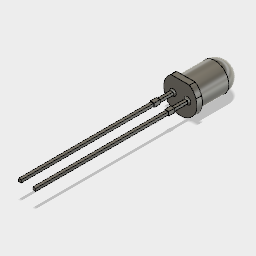
Diode with cutout v1 (Autodesk Fusion 360 design; units mm, degrees)
Autodesk Fusion 360 part; units mm, degrees
cylinder "CylinderPrimitive1" add diameter 5 height 0.5 placed x (1, 0, 0) y (0, 1, 0) z (0, 0, 1) at (0, 0, 0) makes body 1
move_body "Move1" bodies 1 to x (1, 0, 0) y (0, 1, 0) z (0, 0, 1) at (-2.2514, 0, -0.3716)
move_face "MoveFace1" by (0, 0, -4.6246) 1 faces at (-3.1377, 0.2321, -0.3716) on bodies 1
sphere "SpherePrimitive1" add diameter 5 placed x (1, 0, 0) y (0, 0, -1) z (0, 1, 0) at (-2.2514, 0, -4.9962) bodies 1
cylinder "CylinderPrimitive2" add diameter 5.9 height 1 placed x (1, 0, 0) y (0, 1, 0) z (0, 0, 1) at (6.2604, 2.0707, 0.1284) separate body makes body 2
move_body "Move2" bodies 2 to x (1, 0, 0) y (0, 1, 0) z (0, 0, 1) at (-8.4959, 0, 0)
move_body "Move3" bodies 2 to x (1, 0, 0) y (0, 1, 0) z (0, 0, 1) at (-0.0535, -1.9528, 0)
cylinder "CylinderPrimitive3" add diameter 5.906 height 1 placed x (1, 0, 0) y (0, 1, 0) z (0, 0, 1) at (-2.2514, 0, 0.1284) bodies 1
combine "Combine1" operation add target body 2 tool bodies 1
sphere "SpherePrimitive2" add diameter 1.5 placed x (1, 0, 0) y (0, 0, -1) z (0, 1, 0) at (-3.6739, 0, 2.7436) separate body makes body 3
move_body "Move4" bodies 3 to x (1, 0, 0) y (0, 1, 0) z (0, 0, 1) at (0.1106, 0, -2.102)
copy_body "CopyPasteBodies1" bodies 3 makes body 4
move_body "Move5" bodies 4 to x (1, 0, 0) y (0, 1, 0) z (0, 0, 1) at (2.5576, 0, 0.0489)
combine "Combine2" operation add target body 2 tool bodies 3 4
box "BoxPrimitive1" add length 27 width 0.5 height 0.5 placed x (0, 0, 1) y (1, 0, 0) z (0, 1, 0) at (-3.8323, 0, 1.4941) separate body makes body 5
move_body "Move6" bodies 5 to x (1, 0, 0) y (0, 1, 0) z (0, 0, 1) at (-0.0201, -0.2558, -0.183)
move_body "Move7" bodies 5 to x (1, 0, 0) y (0, 1, 0) z (0, 0, 1) at (0.0552, 0, 0.0276)
copy_body "CopyPasteBodies2" bodies 5 makes body 6
move_body "Move8" bodies 6 to x (1, 0, 0) y (0, 1, 0) z (0, 0, 1) at (2.5829, 0, 0)
move_body "Move9" bodies 5 to x (1, 0, 0) y (0, 1, 0) z (0, 0, 1) at (-0.0257, 0.0152, 0)
move_body "Move10" bodies 6 to x (1, 0, 0) y (0, 1, 0) z (0, 0, 1) at (-0.0376, -0.0083, 0)
combine "Combine3" operation add target body 2 tool bodies 5 6
box "BoxPrimitive2" add length 1.0945 width 0.7036 height 0.7 placed x (0, 0, -1) y (-1, 0, 0) z (0, 1, 0) at (1.6805, 0, 5.7753) separate body makes body 7
move_body "Move11" bodies 7 to x (1, 0, 0) y (0, 1, 0) z (0, 0, 1) at (-4.9056, -0.3489, -0.9674)
copy_body "CopyPasteBodies3" bodies 7 makes body 8
move_body "Move12" bodies 8 to x (1, 0, 0) y (0, 1, 0) z (0, 0, 1) at (2.5717, -0.0181, 0)
combine "Combine4" operation add target body 2 tool bodies 7 8
move_body "Move13" bodies 2 to x (1, 0, 0) y (0, 1, 0) z (0, 0, 1) at (-11.8911, -2.3552, 0)
box "BoxPrimitive3" add length 1.4648 width 5.1413 height -4 placed x (0, 1, 0) y (-1, 0, 0) z (0, 0, 1) at (-11.1846, 0.1525, 0) separate body makes body 9
move_body "Move14" bodies 9 to x (1, 0, 0) y (0, 1, 0) z (0, 0, 1) at (-0.3457, 0.0546, 2)
combine "Combine5" operation cut target body 2 tool bodies 9
